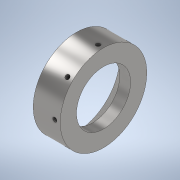
# Autodesk Inventor part: ODSY-0003-101
Saved by Autodesk Inventor 2021 (Build 250183000, 183)
## iProperties
Company: ERPL
Created: 2021-10-20
Material: Stainless Steel
Document SubType Name: Modeling
Designer: ALEX CLAY
Density: 8 g/cm^3
Appearance: Semi-Polished
Mass: 891.546 g
Surface Area: 261.791 cm^2
Volume: 111.443 cm^3
Project: ODYSSEY
Description: NOZZLE HOLDER
Part Number: ODSY-0003-101
Author: ALEX CLAY
Revision Number: 00
Autodesk Inventor part; units mm, degrees
ref_plane "YZ Plane" through (0, 0, 0) normal (1, 0, 0) x (0, 1, 0)
ref_plane "XZ Plane" through (0, 0, 0) normal (0, 1, 0) x (-1, 0, 0)
derived "Rao Nozzle.ipt"
sketch "Sketch1" plane through (0, 0, 0) normal (0, 0, 1) x (1, 0, 0)
  arc A0 (-10.3341, 13.9464) -> (0, 9.525) centre (0, 23.8125) ccw
  arc A1 (0, 9.525) -> (1.2445, 9.7444) centre (0, 13.1635) ccw
  line L0 (-7.4701, 9.525) -> (9.7854, 9.525) construction
  line L1 (-10.3341, 13.9464) -> (-37.5801, 42.4849)
  arc A2 (46.7269, 21.0845) -> (1.2445, 9.7444) centre (77.9324, -200.954) ccw
  line L2 (1.2445, 9.7444) -> (30.761, 20.4876) construction
  line L3 (46.7269, 21.0845) -> (89.89, 27.1507) construction
  line L4 (46.7269, 21.0845) -> (95.911, 21.0845) construction
  line L5 (-42.1731, 50.8) -> (46.7269, 50.8)
  line L6 (46.7269, 50.8) -> (46.7269, 21.0845)
  line L7 (-72.1769, 0) -> (123.9257, 0)
  arc A3 (-37.5801, 42.4849) -> (-42.1731, 44.45) centre (-42.1731, 38.1) ccw
  line L8 (-42.1731, 44.45) -> (-42.1731, 50.8)
  line L9 (46.7269, 31.75) -> (34.0269, 31.75)
  line L10 (34.0269, 31.75) -> (14.9769, 50.8)
  point P0 (0, 0)
revolve "Revolution1" add sketch "Sketch1" angle 360 about axis through (-10, 0, 0) along (1, 0, 0) contours L9 L10 L5 L6
ref_plane "Work Plane1" through (30.8519, 0, 50.8) normal (0, 0, 1) x (1, 0, 0)
sketch "Sketch2" plane through (30.8519, 0, 50.8) normal (0, 0, 1) x (1, 0, 0)
  line L0 (15.875, -50.8) -> (15.875, 50.8) projected
  point P0 (-30.8519, 0)
  point P1 (9.525, 0)
  dimension "d2" = 6.35
  constraints: 1 horizontal alignment
  measures "d2" distance from line of L0 point (9.525, 0)
hole "Hole1" at (40.3769, 0, 50.8) direction (0, 0, -1) diameter 4.9784 depth 12.7 thread size "1/4-20 UNC" class "2B" standard "ANSI Unified Screw Threads"
pattern_circular "Circular Pattern1" count 8 over 360 about axis through (30.8519, 0, 0) along (1, 0, 0) of "Hole1"
body "Solid1"
